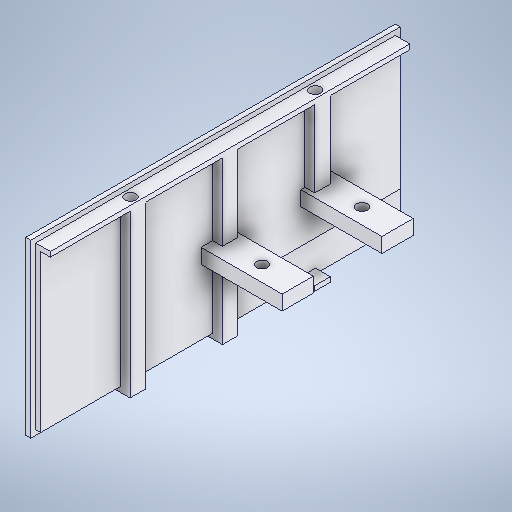
# Autodesk Inventor part: leftwall
Saved by Autodesk Inventor 2025 (Build 290162000, 162)
## iProperties
Created: 2025-05-12
Part Number: leftwall
Material: Generic
Document SubType Name: Modeling
Designer: ethan
Density: 1 g/cm^3
Appearance: PTFE
Author: ethan
Autodesk Inventor part; units mm, degrees
ref_plane "YZ Plane" through (0, 0, 0) normal (1, 0, 0) x (0, 1, 0)
ref_plane "XZ Plane" through (0, 0, 0) normal (0, 1, 0) x (-1, 0, 0)
ref_plane "XY Plane" through (0, 0, 0) normal (0, 0, 1) x (1, 0, 0)
sketch "Sketch1" plane through (0, 0, 0) normal (1, 0, 0) x (0, 1, 0)
  line L0 (0, 0) -> (69.85, 0)
  line L1 (69.85, 0) -> (69.85, -150.4)
  line L2 (69.85, -150.4) -> (0, -150.4)
  line L3 (0, -150.4) -> (0, 0)
  dimension "d0" = 69.85
  dimension "d1" = 150.4
  constraints: 8 end point, 2 parallel, 1 horizontal, 1 perpendicular
  measures "d0" distance of L1.end L2.end
  measures "d1" distance of L0.end L1.end
extrude "Extrusion1" add sketch "Sketch1" along normal blind 2
sketch "Sketch2" plane through (2, 0, 0) normal (1, 0, 0) x (0, 0, -1)
  line L0 (150.4, 0) -> (150.4, 69.85) projected
  line L1 (150.4, 69.85) -> (0, 69.85) projected
  line L2 (0, 69.85) -> (0, 0) projected
  line L3 (0, 0) -> (150.4, 0) projected
  line L4 (150.4, 69.85) -> (148.4, 69.85)
  line L5 (148.4, 69.85) -> (148.4, 0)
  line L6 (148.4, 0) -> (150.4, 0)
  line L7 (150.4, 0) -> (150.4, 69.85)
  line L8 (0, 69.85) -> (2, 69.85)
  line L9 (2, 69.85) -> (2, 0)
  line L10 (2, 0) -> (0, 0)
  line L11 (0, 0) -> (0, 69.85)
  line L12 (0, 0) -> (150.4, 0)
  line L13 (150.4, 0) -> (150.4, 2)
  line L14 (150.4, 2) -> (0, 2)
  line L15 (0, 2) -> (0, 0)
  point P0 (2, 2)
  point P1 (148.4, 2)
  dimension "d4" = 2
  dimension "d5" = 2
  dimension "d6" = 2
  constraints: 24 end point, 6 parallel, 3 horizontal, 3 perpendicular, 3 point on line
  measures "d4" distance of L6.end L5.end
  measures "d5" distance of L9.end L10.end
  measures "d6" distance of L13.end L12.end
extrude "Extrusion2" add sketch "Sketch2" along normal blind 2 contours L14 L9 L1 L5
sketch "Sketch3" plane through (4, 0, 0) normal (1, 0, 0) x (0, 0, -1)
  line L0 (150.4, 0) -> (150.4, 69.85) projected
  line L1 (0, 0) -> (150.4, 0) projected
  line L2 (0, 69.85) -> (0, 0) projected
  line L3 (150.4, 69.85) -> (0, 69.85) projected
  line L4 (0, 69.85) -> (75.2, 69.85) construction
  line L5 (75.2, 69.85) -> (75.2, 0) construction
  line L6 (75.2, 0) -> (0, 0) construction
  line L7 (0, 0) -> (0, 69.85) construction
  line L8 (0, 0) -> (150.4, 0) construction
  line L9 (0, 0) -> (37.6, 0) construction
  line L10 (37.6, 0) -> (37.6, 69.85) construction
  line L11 (37.6, 69.85) -> (0, 69.85) construction
  line L12 (0, 69.85) -> (0, 0) construction
  line L13 (150.4, 0) -> (150.4, 69.85) construction
  line L14 (75.2, 69.85) -> (150.4, 69.85) construction
  line L15 (150.4, 69.85) -> (150.4, 0) construction
  line L16 (150.4, 0) -> (75.2, 0) construction
  line L17 (75.2, 0) -> (75.2, 69.85) construction
  line L18 (75.2, 0) -> (112.8, 0) construction
  line L19 (112.8, 0) -> (112.8, 69.85) construction
  line L20 (112.8, 69.85) -> (75.2, 69.85) construction
  line L21 (75.2, 69.85) -> (75.2, 0) construction
  line L22 (34.425, 0) -> (34.425, 69.85) construction
  line L23 (34.425, 69.85) -> (40.775, 69.85) construction
  line L24 (40.775, 69.85) -> (40.775, 0) construction
  line L25 (40.775, 0) -> (34.425, 0) construction
  line L26 (34.425, 0) -> (40.775, 69.85) construction
  line L27 (34.425, 69.85) -> (40.775, 0) construction
  line L28 (72.025, 0) -> (72.025, 69.85) construction
  line L29 (72.025, 69.85) -> (78.375, 69.85) construction
  line L30 (78.375, 69.85) -> (78.375, 0) construction
  line L31 (78.375, 0) -> (72.025, 0) construction
  line L32 (72.025, 0) -> (78.375, 69.85) construction
  line L33 (72.025, 69.85) -> (78.375, 0) construction
  line L34 (109.625, 0) -> (109.625, 69.85) construction
  line L35 (109.625, 69.85) -> (115.975, 69.85) construction
  line L36 (115.975, 69.85) -> (115.975, 0) construction
  line L37 (115.975, 0) -> (109.625, 0) construction
  line L38 (109.625, 0) -> (115.975, 69.85) construction
  line L39 (109.625, 69.85) -> (115.975, 0) construction
  line L40 (34.425, 69.85) -> (40.775, 69.85)
  line L41 (40.775, 69.85) -> (40.775, 0)
  line L42 (40.775, 0) -> (34.425, 0)
  line L43 (34.425, 0) -> (34.425, 69.85)
  line L44 (72.025, 0) -> (78.375, 0)
  line L45 (78.375, 0) -> (78.375, 69.85)
  line L46 (78.375, 69.85) -> (72.025, 69.85)
  line L47 (72.025, 69.85) -> (72.025, 0)
  line L48 (109.625, 69.85) -> (115.975, 69.85)
  line L49 (115.975, 69.85) -> (115.975, 0)
  line L50 (115.975, 0) -> (109.625, 0)
  line L51 (109.625, 0) -> (109.625, 69.85)
  point P0 (37.6, 34.925)
  point P1 (75.2, 34.925)
  point P2 (112.8, 34.925)
  dimension "d9" = 6.35
  dimension "d10" = 6.35
  dimension "d11" = 6.35
  constraints: 92 end point, 21 parallel, 12 midpoint, 12 perpendicular, 7 horizontal
  measures "d9" distance of L22.end L23.end
  measures "d10" distance of L28.end L29.end
  measures "d11" distance of L34.end L35.end
extrude "Extrusion3" add sketch "Sketch3" along normal blind 4 contours L1 L51 L3 L49 | L1 L47 L3 L45 | L1 L43 L3 L41
sketch "Sketch4" plane through (0, 69.85, 0) normal (0, 1, 0) x (1, 0, 0)
  line L0 (0, 150.4) -> (0, 0) projected
  line L1 (0, 150.4) -> (0, 0) construction
  line L2 (0, 0) -> (2, 0) construction
  line L3 (2, 2) -> (2, 0) construction
  line L4 (2, 2) -> (4, 2) construction
  line L5 (4, 34.425) -> (4, 2) construction
  line L6 (4, 34.425) -> (8, 34.425) construction
  line L7 (8, 40.775) -> (8, 34.425) construction
  line L8 (4, 40.775) -> (8, 40.775) construction
  line L9 (4, 72.025) -> (4, 40.775) construction
  line L10 (4, 72.025) -> (8, 72.025) construction
  line L11 (8, 78.375) -> (8, 72.025) construction
  line L12 (4, 78.375) -> (8, 78.375) construction
  line L13 (4, 109.625) -> (4, 78.375) construction
  line L14 (4, 109.625) -> (8, 109.625) construction
  line L15 (8, 115.975) -> (8, 109.625) construction
  line L16 (4, 115.975) -> (8, 115.975) construction
  line L17 (4, 148.4) -> (4, 115.975) construction
  line L18 (2, 148.4) -> (4, 148.4) construction
  line L19 (2, 150.4) -> (2, 148.4) construction
  line L20 (0, 150.4) -> (2, 150.4) construction
  line L21 (2, 0) -> (0, 0)
  line L22 (0, 0) -> (0, 150.4)
  line L23 (0, 150.4) -> (2, 150.4)
  line L24 (2, 150.4) -> (2, 0)
  line L25 (2, 0) -> (8, 0)
  line L26 (8, 0) -> (8, 150.4)
  line L27 (8, 150.4) -> (2, 150.4)
  line L28 (2, 150.4) -> (2, 0)
  constraints: 16 end point, 4 parallel, 2 horizontal, 2 perpendicular
extrude "Extrusion4" cut sketch "Sketch4" against normal blind 2 contours L27 L26 L25 L24
sketch "Sketch5" plane through (0, 67.85, 0) normal (0, 1, 0) x (1, 0, 0)
  line L0 (4, 115.975) -> (8, 115.975) projected
  line L1 (4, 148.4) -> (4, 115.975) projected
  line L2 (2, 148.4) -> (4, 148.4) projected
  line L3 (2, 2) -> (2, 148.4) projected
  line L4 (4, 2) -> (2, 2) projected
  line L5 (4, 34.425) -> (4, 2) projected
  line L6 (8, 34.425) -> (4, 34.425) projected
  line L7 (8, 40.775) -> (8, 34.425) projected
  line L8 (4, 40.775) -> (8, 40.775) projected
  line L9 (4, 72.025) -> (4, 40.775) projected
  line L10 (8, 72.025) -> (4, 72.025) projected
  line L11 (8, 78.375) -> (8, 72.025) projected
  line L12 (4, 78.375) -> (8, 78.375) projected
  line L13 (4, 109.625) -> (4, 78.375) projected
  line L14 (8, 109.625) -> (4, 109.625) projected
  line L15 (8, 115.975) -> (8, 109.625) projected
  line L16 (2, 2) -> (4, 2) projected
  line L17 (2, 2) -> (8, 2)
  line L18 (8, 2) -> (8, 148.4)
  line L19 (8, 148.4) -> (2, 148.4)
  line L20 (2, 148.4) -> (2, 2)
  point P0 (0, 0)
  point P1 (4, 2)
  constraints: 8 end point, 2 parallel, 1 horizontal, 1 perpendicular
extrude "Extrusion5" add sketch "Sketch5" against normal blind 2 contours L1 L19 L18 L0 | L18 L12 L13 L14 | L18 L8 L9 L10 | L5 L6 L18 L17
sketch "Sketch6" plane through (4, 0, 0) normal (1, 0, 0) x (0, 0, -1)
  line L0 (2, 67.85) -> (148.4, 67.85) construction
  line L1 (2, 67.85) -> (2, 65.85) construction
  line L2 (34.425, 65.85) -> (2, 65.85) construction
  line L3 (34.425, 65.85) -> (34.425, 0) construction
  line L4 (34.425, 0) -> (40.775, 0) construction
  line L5 (40.775, 0) -> (40.775, 65.85) construction
  line L6 (72.025, 65.85) -> (40.775, 65.85) construction
  line L7 (72.025, 65.85) -> (72.025, 0) construction
  line L8 (72.025, 0) -> (78.375, 0) construction
  line L9 (78.375, 0) -> (78.375, 65.85) construction
  line L10 (109.625, 65.85) -> (78.375, 65.85) construction
  line L11 (109.625, 65.85) -> (109.625, 0) construction
  line L12 (109.625, 0) -> (115.975, 0) construction
  line L13 (115.975, 0) -> (115.975, 65.85) construction
  line L14 (148.4, 65.85) -> (115.975, 65.85) construction
  line L15 (148.4, 67.85) -> (148.4, 65.85) construction
  line L16 (109.625, 65.85) -> (78.375, 65.85) construction
  line L17 (78.375, 65.85) -> (78.375, 2) construction
  line L18 (78.375, 2) -> (109.625, 2) construction
  line L19 (109.625, 2) -> (109.625, 65.85) construction
  line L20 (148.4, 65.85) -> (115.975, 65.85) construction
  line L21 (115.975, 65.85) -> (115.975, 2) construction
  line L22 (115.975, 2) -> (148.4, 2) construction
  line L23 (148.4, 2) -> (148.4, 65.85) construction
  line L24 (72.025, 65.85) -> (40.775, 65.85) construction
  line L25 (40.775, 65.85) -> (40.775, 2) construction
  line L26 (40.775, 2) -> (72.025, 2) construction
  line L27 (72.025, 2) -> (72.025, 65.85) construction
  line L28 (78.375, 2) -> (78.375, 28.67) construction
  line L29 (94, 28.67) -> (114.32, 28.67)
  line L30 (114.32, 28.67) -> (73.68, 28.67)
  line L31 (73.68, 28.67) -> (67.33, 28.67)
  line L32 (67.33, 28.67) -> (80.03, 28.67)
  line L33 (80.03, 28.67) -> (80.03, 34.67)
  line L34 (80.03, 34.67) -> (67.33, 34.67)
  line L35 (67.33, 34.67) -> (67.33, 28.67)
  line L36 (114.32, 28.67) -> (120.67, 28.67)
  line L37 (120.67, 28.67) -> (107.97, 28.67)
  line L38 (107.97, 28.67) -> (107.97, 34.67)
  line L39 (107.97, 34.67) -> (120.67, 34.67)
  line L40 (120.67, 34.67) -> (120.67, 28.67)
  point P0 (0, 0)
  dimension "d18" = 26.67
  dimension "d31" = 20.32
  dimension "d32" = 40.64
  dimension "d33" = 6.35
  dimension "d34" = 12.7
  dimension "d35" = 6
  dimension "d36" = 6.35
  dimension "d37" = 12.7
  dimension "d38" = 6
  constraints: 26 end point, 4 parallel, 4 point on line, 3 horizontal, 2 perpendicular
  measures "d18" distance of L17.end L28.end
  measures "d31" distance of L29.start L29.end
  measures "d32" distance of L29.end L30.end
  measures "d33" distance of L30.end L31.end
  measures "d34" distance of L34.end L33.end
  measures "d35" distance of L33.end L32.end
  measures "d36" distance of L29.end L36.end
  measures "d37" distance of L38.end L39.end
  measures "d38" distance of L37.end L38.end
extrude "Extrusion6" add sketch "Sketch6" along normal blind 33.02
sketch "Sketch12" plane through (4, 34.67, -67.33) normal (0, 1, 0) x (1, 0, 0)
  line L0 (4, 11.045) -> (0, 11.045) construction
  line L1 (4, 4.695) -> (4, 11.045) construction
  line L2 (0, 4.695) -> (4, 4.695) construction
  line L3 (0, 0) -> (0, 4.695) construction
  line L4 (0, 0) -> (33.02, 0) construction
  line L5 (33.02, 12.7) -> (33.02, 0) construction
  line L6 (0, 12.7) -> (33.02, 12.7) construction
  line L7 (0, 11.045) -> (0, 12.7) construction
  line L8 (4, 48.645) -> (0, 48.645) construction
  line L9 (4, 42.295) -> (4, 48.645) construction
  line L10 (0, 42.295) -> (4, 42.295) construction
  line L11 (0, 40.64) -> (0, 42.295) construction
  line L12 (0, 40.64) -> (33.02, 40.64) construction
  line L13 (33.02, 53.34) -> (33.02, 40.64) construction
  line L14 (0, 53.34) -> (33.02, 53.34) construction
  line L15 (0, 48.645) -> (0, 53.34) construction
  line L16 (4, 4.695) -> (4, -26.555) construction
  line L17 (4, 4.695) -> (33.02, 4.695) construction
  line L18 (33.02, 4.695) -> (33.02, 0) construction
  line L19 (33.02, 0) -> (4, 0) construction
  line L20 (4, 0) -> (4, 4.695) construction
  circle A0 centre (18.51, 6.35) radius 2.25 construction
  line L21 (4, 48.645) -> (33.02, 48.645) construction
  circle A1 centre (18.51, 46.99) radius 2.25 construction
  circle A2 centre (18.51, 6.35) radius 2.25
  circle A3 centre (18.51, 46.99) radius 2.25
  point P0 (-4, -67.33)
  dimension "d39" = 4.5
  dimension "d40" = 4.5
  constraints: 10 end point, 4 centre point, 2 coincident, 2 concentric, 2 parallel, 2 perpendicular, 1 horizontal, 1 point on line
  measures "d39" diameter of A0
  measures "d40" diameter of A1
extrude "Extrusion10" cut sketch "Sketch12" against normal blind 5
sketch "Sketch13" plane through (8, 0, 0) normal (1, 0, 0) x (0, 0, -1)
  line L0 (120.67, 28.67) -> (115.975, 28.67) construction
  line L1 (115.975, 28.67) -> (115.975, 2) construction
  line L2 (115.975, 2) -> (148.4, 2) construction
  line L3 (148.4, 2) -> (148.4, 65.85) construction
  line L4 (148.4, 65.85) -> (115.975, 65.85) construction
  line L5 (115.975, 65.85) -> (115.975, 34.67) construction
  line L6 (115.975, 34.67) -> (120.67, 34.67) construction
  line L7 (120.67, 34.67) -> (120.67, 28.67) construction
  line L8 (115.975, 28.67) -> (109.625, 28.67) construction
  line L9 (109.625, 28.67) -> (109.625, 0) construction
  line L10 (109.625, 0) -> (115.975, 0) construction
  line L11 (115.975, 0) -> (115.975, 28.67) construction
  line L12 (78.375, 2) -> (109.625, 2) projected
  line L13 (115.975, 28.67) -> (109.625, 28.67)
  line L14 (109.625, 28.67) -> (109.625, 2)
  line L15 (109.625, 2) -> (115.975, 2)
  line L16 (115.975, 2) -> (115.975, 28.67)
  point P0 (0, 0)
  constraints: 8 end point, 2 parallel, 1 horizontal, 1 perpendicular
extrude "Extrusion11" cut sketch "Sketch13" against normal up to surface (4 mm away)
sketch "Sketch14" plane through (4, 0, 0) normal (-1, 0, 0) x (0, 0, 1)
  line L0 (-109.625, 2) -> (-115.975, 2) projected
  line L1 (-115.975, 0) -> (-115.975, 2) projected
  line L2 (-109.625, 0) -> (-115.975, 0) projected
  line L3 (-109.625, 2) -> (-109.625, 0) projected
  line L4 (-72.025, 2) -> (-78.375, 2) projected
  line L5 (-78.375, 0) -> (-78.375, 2) projected
  line L6 (-72.025, 0) -> (-78.375, 0) projected
  line L7 (-72.025, 2) -> (-72.025, 0) projected
  line L8 (-34.425, 2) -> (-40.775, 2) projected
  line L9 (-40.775, 0) -> (-40.775, 2) projected
  line L10 (-34.425, 0) -> (-40.775, 0) projected
  line L11 (-34.425, 2) -> (-34.425, 0) projected
  point P0 (0, 0)
extrude "Extrusion12" add sketch "Sketch14" along normal blind 2
sketch "Sketch15" plane through (0, 67.85, 0) normal (0, 1, 0) x (1, 0, 0)
  line L0 (8, 2) -> (8, 148.4) construction
  line L1 (2, 148.4) -> (8, 148.4) construction
  line L2 (2, 2) -> (2, 148.4) construction
  line L3 (8, 2) -> (2, 2) construction
  line L4 (8, 109.625) -> (8, 115.975) construction
  line L5 (8, 148.4) -> (8, 115.975) construction
  line L6 (8, 2) -> (8, 148.4) construction
  line L7 (8, 34.425) -> (8, 2) construction
  line L8 (8, 34.425) -> (8, 40.775) construction
  line L9 (8, 72.025) -> (8, 40.775) construction
  line L10 (8, 72.025) -> (8, 78.375) construction
  line L11 (8, 109.625) -> (8, 78.375) construction
  line L12 (8, 34.425) -> (4, 34.425) construction
  line L13 (8, 34.425) -> (2, 34.425) construction
  line L14 (2, 34.425) -> (2, 40.775) construction
  line L15 (2, 40.775) -> (8, 40.775) construction
  line L16 (8, 40.775) -> (8, 34.425) construction
  line L17 (8, 109.625) -> (2, 109.625) construction
  line L18 (2, 109.625) -> (2, 115.975) construction
  line L19 (2, 115.975) -> (8, 115.975) construction
  line L20 (8, 115.975) -> (8, 109.625) construction
  circle A0 centre (5, 37.6) radius 2.25 construction
  circle A1 centre (5, 37.6) radius 2.25
  circle A2 centre (5, 112.8) radius 2.25
  point P0 (0, 0)
  dimension "d47" = 4.5
  dimension "d48" = 4.5
  constraints: 16 end point, 4 parallel, 3 centre point, 2 horizontal, 2 perpendicular, 2 point on line, 1 coincident, 1 concentric
  measures "d47" diameter of A0
  measures "d48" diameter of A2
extrude "Extrusion13" cut sketch "Sketch15" against normal blind 5
sketch "Sketch16" plane through (4, 0, 0) normal (1, 0, 0) x (0, 0, -1)
  line L0 (107.97, 28.67) -> (120.67, 28.67) construction
  line L1 (107.97, 28.67) -> (107.97, 34.67) construction
  line L2 (107.97, 34.67) -> (109.625, 34.67) construction
  line L3 (109.625, 34.67) -> (109.625, 65.85) construction
  line L4 (109.625, 65.85) -> (78.375, 65.85) construction
  line L5 (78.375, 65.85) -> (78.375, 34.67) construction
  line L6 (78.375, 34.67) -> (80.03, 34.67) construction
  line L7 (80.03, 34.67) -> (80.03, 28.67) construction
  line L8 (80.03, 28.67) -> (78.375, 28.67) construction
  line L9 (78.375, 28.67) -> (78.375, 2) construction
  line L10 (78.375, 2) -> (109.625, 2) construction
  line L11 (109.625, 2) -> (115.975, 2) construction
  line L12 (115.975, 2) -> (148.4, 2) construction
  line L13 (148.4, 2) -> (148.4, 65.85) construction
  line L14 (148.4, 65.85) -> (115.975, 65.85) construction
  line L15 (115.975, 65.85) -> (115.975, 34.67) construction
  line L16 (115.975, 34.67) -> (120.67, 34.67) construction
  line L17 (120.67, 34.67) -> (120.67, 28.67) construction
  line L18 (148.4, 2) -> (78.375, 2) construction
  line L19 (78.375, 2) -> (78.375, 14.7) construction
  line L20 (78.375, 14.7) -> (148.4, 14.7) construction
  line L21 (148.4, 14.7) -> (148.4, 2) construction
  line L22 (115.975, 2) -> (148.4, 2) projected
  line L23 (78.375, 14.7) -> (148.4, 14.7)
  line L24 (148.4, 14.7) -> (148.4, 2)
  line L25 (148.4, 2) -> (78.375, 2)
  line L26 (78.375, 2) -> (78.375, 14.7)
  point P0 (0, 0)
  dimension "d51" = 12.7
  constraints: 16 end point, 4 parallel, 2 horizontal, 2 perpendicular, 1 point on line
  measures "d51" distance of L18.end L19.end
extrude "Extrusion14" cut sketch "Sketch16" against normal up to surface (2 mm away)
body "Solid1"
